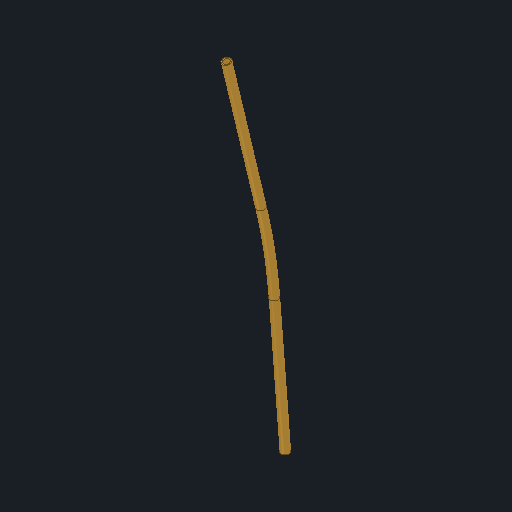
# Autodesk Inventor part: prop_shaft
Saved by Autodesk Inventor 2023 (Build 270158030, 158C)
## iProperties
Created: 2022-04-18
Part Number: prop_shaft
Material: Generic
Document SubType Name: Modeling
Designer: kardo
Density: 1 g/cm^3
Appearance: Brass - Prop shaft
Mass: 2.97565 g
Surface Area: 75.2146 cm^2
Volume: 2.97565 cm^3
Author: kardo
Autodesk Inventor part; units mm, degrees
ref_plane "YZ Plane" through (0, 0, 0) normal (1, 0, 0) x (0, 1, 0)
ref_plane "XZ Plane" through (0, 0, 0) normal (0, 1, 0) x (-1, 0, 0)
ref_plane "XY Plane" through (0, 0, 0) normal (0, 0, 1) x (1, 0, 0)
derived "stencil_frame.ipt"
sketch "sk_drivetrain_profile" plane through (6, 0, 0) normal (1, 0, 0) x (0, 1, 0)
  line L0 (-529.1844, 0) -> (410.1064, 0) construction
  line L1 (-345, 3089.1136) -> (-345, -1866.0023) construction
  line L2 (0, 3089.1136) -> (0, -1866.0023) construction
  line L3 (-133.502, 53.1159) -> (-126.9655, 25.8896)
  line L4 (-377, 0) -> (-313.1973, 5.0214)
  line L5 (-130.2338, 39.5028) -> (-226.4223, 16.4099)
  line L6 (-283.6394, 7.3476) -> (-254.6742, 9.6272) construction
  line L7 (-254.6742, 9.6272) -> (-226.4223, 16.4099) construction
  line L8 (-126.9655, 25.8896) -> (-126.9655, 20.8896) construction
  line L9 (-313.1973, 5.0214) -> (-283.6394, 7.3476)
  line L10 (-844.2225, 3013.4797) -> (331.7536, -1884.8132) construction
  line L11 (-227.0708, 19.1113) -> (-130.8823, 42.2041) construction
  line L12 (-129.5852, 36.8014) -> (-225.7737, 13.7086) construction
  line L13 (-227.0708, 19.1113) -> (-225.7737, 13.7086) construction
  spline S0 degree 2 poles (-283.6394, 7.3476) (-254.6742, 9.6272) (-226.4223, 16.4099) knots 1 1 1 2 2 2
  line L14 (0, 21.3303) -> (-241.5001, 18.9703) construction
  line L15 (-48.9013, 21.6524) -> (-303.0379, 19.169) construction
  point P0 (0, 0)
  point P1 (-214.6653, 19.2325)
  point P2 (-202.2599, 19.3538)
  point P3 (-198.7861, 20.1877)
ref_plane "plane_motor_mount" through (0, -120.75, 0) normal (0, 0.9723699, 0.2334454) x (-1, 0, 0)
sketch "sk_prop_shaft_profile" plane through (0, -120.75, 0) normal (0, 0.9723699, 0.2334454) x (-1, 0, 0)
  circle A0 centre (-6, 40.6252) radius 2.7781
  point P0 (0, -28.1885)
  dimension "d1" = 5.5563
  constraints: 1 centre point, 1 coincident
  measures "d1" diameter of A0
derived "parameters_powertrain.ipt"
sweep "Sweep1" add profiles "sk_prop_shaft_profile" path "sk_drivetrain_profile" path curves L5 S0 L9 L4
shell "Shell1" thickness 0.7937 removed faces 2 at (5.8387, -377.04, 0.5088) at (6.6932, -130.3771, 40.0999)
equation "\"d1\" = prop_shaft_sleeve_od"
equation "\"prop_shaft_sleeve_od\" = 5.55625"
body "Solid1"
